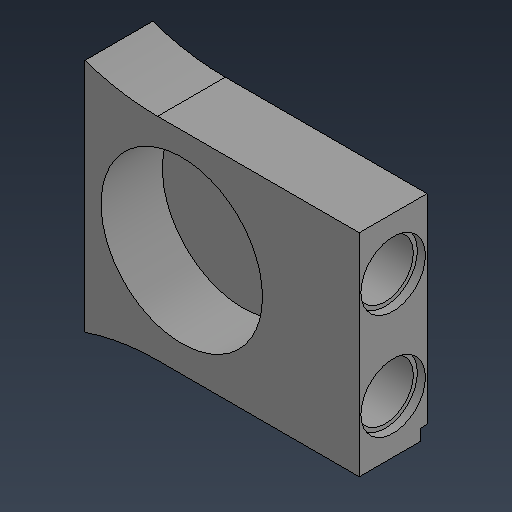
# Autodesk Inventor part: BearigHoldRight
Saved by Autodesk Inventor 2026.2 (Build 302298010, 298A)
## iProperties
Created: 2026-04-04
Part Number: BearigHoldRight
Material: Generic
Document SubType Name: Modeling
Designer: szymo
Density: 1 g/cm^3
Appearance: Default(1)
Author: szymo
Autodesk Inventor part; units mm, degrees
ref_plane "YZ Plane" through (0, 0, 0) normal (1, 0, 0) x (0, 1, 0)
ref_plane "XZ Plane" through (0, 0, 0) normal (0, 1, 0) x (-1, 0, 0)
ref_plane "XY Plane" through (0, 0, 0) normal (0, 0, 1) x (1, 0, 0)
sketch "Sketch1" plane through (0, 0, 0) normal (0, 0, 1) x (1, 0, 0)
  circle A0 centre (-14.5, 55.2958) radius 13.85 projected
  circle A1 centre (-14.5, 55.2958) radius 14.5 projected
  circle A2 centre (-14.5, 14.5) radius 13.85 projected
  circle A3 centre (-14.5, 14.5) radius 14.5 projected
  circle A4 centre (-13, 35.0012) radius 5 projected
  line L0 (0, 65.2958) -> (-19, 65.2958)
  line L1 (-19, 65.2958) -> (-19, -1.7042)
  line L2 (-19, -1.7042) -> (0, -1.7042)
  line L3 (0, -1.7042) -> (0, 65.2958)
  line L4 (-2, 65.2958) -> (-2, -1.7042)
  line L5 (-14.5, 41.4458) -> (-2, 41.4458)
  line L6 (-14.5, 40.7958) -> (-2, 40.7958)
  line L7 (-14.5, 28.35) -> (-2, 28.35)
  line L8 (-14.5, 29) -> (-2, 29)
  point P0 (0, 0)
  point P1 (-19, 42.1973)
  point P2 (-19, 27.5986)
  point P3 (-19, 28.284)
  point P4 (-19, 41.5118)
  dimension "d0" = 67
  dimension "d1" = 1
  dimension "d2" = 2
  constraints: 18 end point, 6 perpendicular, 6 point on line, 5 horizontal, 2 parallel, 9 other
  measures "d0" distance of L2.end L0.start
  measures "d1" distance edge to line of A4 L1
  measures "d2" distance between parallel lines of L3 L4
extrude "Extrusion1" add sketch "Sketch1" against normal blind 3.8 contours L5 A1 L1 A0 | L5 L4 L6 A1 | A1 L6 L4 L8 A3 L1 | A3 L7 A2 L1 | L4 L7 A3 L8
ref_plane "Work Plane7" through (0, 0, -3.8) normal (0, 0, -1) x (-1, 0, 0)
sketch "Sketch2" plane through (0, 0, -3.8) normal (0, 0, -1) x (-1, 0, 0)
  circle A0 centre (8.5216, 9.2187) radius 1.0564 projected
  circle A1 centre (20.7784, 19.5033) radius 1.0564 projected
  circle A2 centre (14.65, 14.361) radius 5 projected
  circle A3 centre (14.65, 14.361) radius 14 projected
  circle A4 centre (14.65, 14.361) radius 14.7 projected
  line L0 (2, 41.4458) -> (2, 28.35) projected
  line L1 (2, 28.35) -> (14.5, 28.35) projected
  arc A5 (19, 27.5986) -> (14.5, 28.35) centre (14.5, 14.5) ccw projected
  line L2 (19, 27.5986) -> (19, 42.1973) projected
  arc A6 (14.5, 41.4458) -> (19, 42.1973) centre (14.5, 55.2958) ccw projected
  line L3 (14.5, 41.4458) -> (2, 41.4458) projected
  circle A7 centre (13, 35.0012) radius 5 projected
  line L4 (14.5, 29.0603) -> (2, 29.0603)
  line L5 (2, 41.4458) -> (2, 28.35) projected
  line L6 (14.5, 29.0603) -> (14.5, 14.5)
  point P0 (0, 0)
  point P1 (2, 29.0603)
  point P2 (19, 28.4027)
  constraints: 4 end point, 3 perpendicular, 1 horizontal, 1 point on line, 2 other
extrude "Extrusion4" add sketch "Sketch2" along normal blind 0.4 contours A4 L4 L0 L3 A6 L2 | A7
sketch "Sketch3" plane through (-2, 28.35, 0) normal (1, 0, 0) x (0, 0, -1)
  line L0 (0, 0) -> (0, 13.0958) projected
  line L1 (0, 0) -> (3.8, 0) projected
  line L2 (0, 6.5784) -> (4.4, 6.5784)
  line L3 (0, 13.0958) -> (4.4, 6.5784)
  line L4 (4.4, 6.5784) -> (0, 0)
  line L5 (0, 6.5784) -> (2.2, 3.2892)
  line L6 (0, 6.5784) -> (2.2, 9.8371)
  line L7 (0, 13.0958) -> (4.2, 13.0958) projected
  line L8 (3.8, 0.7103) -> (3.8, 0) projected
  line L9 (3.8, 0.7103) -> (4.2, 0.7103) projected
  line L10 (4.2, 13.0958) -> (4.2, 0.7103) projected
  point P0 (0, -28.35)
  point P1 (5.9, 0.65)
  point P2 (5.9, 12.4458)
  dimension "d12" = 6.5784
  constraints: 10 end point, 2 coincident, 2 midpoint, 1 point on line
  measures "d12" distance between parallel lines of L1 L2
hole "Hole1" at (-2, 38.1871, -2.2) at (-2, 31.6392, -2.2) direction (-1, 0, 0) diameter 3.5 depth 4.5 counterbore diameter 4 counterbore depth 0.5
body "Solid1"
